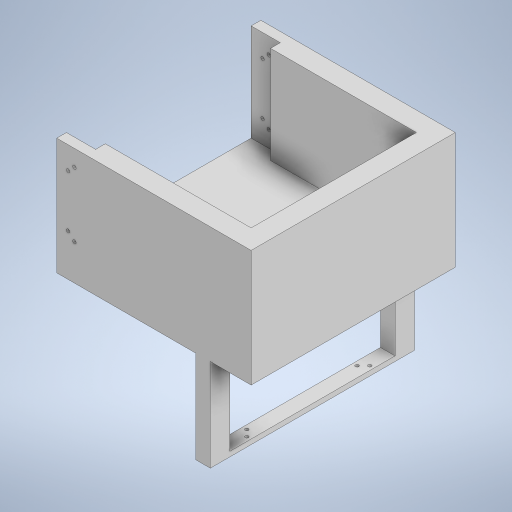
# Autodesk Inventor part: container_front
Saved by Autodesk Inventor 2023 (Build 270158000, 158)
## iProperties
Created: 2022-10-30
Part Number: container_front
Material: Genérico
Document SubType Name: Modeling
Designer: papel
Density: 1 g/cm^3
Appearance: Valor por defecto
Surface Area: 1558.19 cm^2
Author: papel
Autodesk Inventor part; units mm, degrees
ref_plane "YZ Plane" through (0, 0, 0) normal (1, 0, 0) x (0, 1, 0)
ref_plane "XZ Plane" through (0, 0, 0) normal (0, 1, 0) x (-1, 0, 0)
ref_plane "XY Plane" through (0, 0, 0) normal (0, 0, 1) x (1, 0, 0)
sketch "Boceto2" plane through (0, 0, 0) normal (0, 1, 0) x (-1, 0, 0)
  line L0 (7.5, 105) -> (-7.5, 105)
  line L1 (-7.5, 105) -> (-7.5, -105)
  line L2 (-7.5, -105) -> (7.5, -105)
  line L3 (7.5, -105) -> (7.5, 105)
  line L4 (7.5, 105) -> (-7.5, -105) construction
  line L5 (-7.5, 105) -> (7.5, -105) construction
  point P0 (0, 0)
  dimension "d7" = 15
  dimension "d8" = 210
  constraints: 12 end point, 2 midpoint, 2 parallel, 1 horizontal, 1 perpendicular
  measures "d7" distance of L2.end L1.end
  measures "d8" distance of L1.end L0.end
extrude "Extrusión1" add sketch "Boceto2" along normal blind 5
sketch "Boceto3" plane through (0, 5, 0) normal (0, 1, 0) x (1, 0, 0)
  circle A0 centre (3.25, 63.25) radius 1.75
  line L0 (5, 55) -> (-5, 55)
  line L1 (-5, 55) -> (-5, 65)
  line L2 (-5, 65) -> (5, 65)
  line L3 (5, 65) -> (5, 55)
  line L4 (5, 55) -> (-5, 65) construction
  line L5 (-5, 55) -> (5, 65) construction
  circle A1 centre (-3.25, 56.75) radius 1.75
  line L6 (7.5, 105) -> (-7.5, 105) projected
  line L7 (-7.5, 0) -> (3.408, 0)
  line L8 (5, -65) -> (5, -55)
  line L9 (-5, -65) -> (5, -65)
  line L10 (5, -55) -> (-5, -55)
  line L11 (-5, -55) -> (-5, -65)
  line L12 (-5, -55) -> (5, -65) construction
  circle A2 centre (-3.25, -56.75) radius 1.75
  line L13 (5, -55) -> (-5, -65) construction
  circle A3 centre (3.25, -63.25) radius 1.75
  point P0 (0, 0)
  point P1 (-5, 60)
  point P2 (0, 105)
  point P3 (-5, -60)
  dimension "d11" = 3.5
  dimension "d12" = 1.75
  dimension "d13" = 1.75
  dimension "d14" = 1.75
  dimension "d15" = 1.75
  dimension "d16" = 10
  dimension "d17" = 10
  dimension "d19" = 40
  constraints: 26 end point, 7 symmetric about line, 4 centre point, 2 horizontal, 2 midpoint, 2 parallel, 1 perpendicular, 2 other
  measures "d11" diameter of A0
  measures "d12" distance from line of L2 A0.centre
  measures "d13" distance from line of L3 A0.centre
  measures "d14" distance from line of L1 A1.centre
  measures "d15" distance from line of L0 A1.centre
  measures "d16" distance between parallel lines of L0 L2
  measures "d17" distance between parallel lines of L3 L1
  measures "d19" distance from line of point (0, 105) L2
hole "Agujero1" at (3.25, 5, 63.25) at (-3.25, 5, 56.75) at (3.25, 5, -63.25) at (-3.25, 5, -56.75) direction (0, -1, 0) diameter 3.5 end through all
sketch "Boceto4" plane through (0, 5, 0) normal (0, 1, 0) x (1, 0, 0)
  line L0 (-7.5, 105) -> (-7.5, -105) projected
  line L1 (-7.5, -105) -> (7.5, -105)
  line L2 (7.5, -105) -> (7.5, -85)
  line L3 (7.5, -85) -> (-7.5, -85)
  line L4 (-7.5, -85) -> (-7.5, -105)
  line L5 (-7.5, 0) -> (1.0116, 0)
  line L6 (-7.5, -105) -> (-7.5, 105)
  line L7 (-7.5, 105) -> (7.5, 105)
  line L8 (7.5, 105) -> (7.5, 85)
  line L9 (7.5, 85) -> (-7.5, 85)
  line L10 (-7.5, 85) -> (-7.5, 105)
  point P0 (0, 0)
  dimension "d27" = 15
  dimension "d28" = 20
  constraints: 20 end point, 5 symmetric about line, 2 horizontal, 2 parallel, 1 midpoint, 1 perpendicular
  measures "d27" distance of L3.end L2.end
  measures "d28" distance of L2.end L1.end
extrude "Extrusión2" add sketch "Boceto4" along normal blind 90
sketch "Boceto5" plane through (0, 95, 0) normal (0, 1, 0) x (1, 0, 0)
  line L0 (-7.5, -105) -> (7.5, -105) projected
  line L1 (-7.5, -105) -> (49.5, -105)
  line L2 (49.5, -105) -> (49.5, 105)
  line L3 (49.5, 105) -> (-7.5, 105)
  line L4 (-7.5, 105) -> (-7.5, -105)
  line L5 (49.5, -105) -> (-150.5, -105)
  line L6 (-150.5, -105) -> (-150.5, 105)
  line L7 (-150.5, 105) -> (49.5, 105)
  line L8 (49.5, 105) -> (49.5, -105)
  point P0 (0, 0)
  dimension "d31" = 57
  dimension "d32" = 200
  constraints: 16 end point, 4 parallel, 2 horizontal, 2 perpendicular, 1 point on line
  measures "d31" distance of L3.end L2.end
  measures "d32" distance of L6.end L7.end
extrude "Extrusión3" add sketch "Boceto5" along normal blind 120
sketch "Boceto6" plane through (0, 215, 0) normal (0, 1, 0) x (1, 0, 0)
  line L0 (49.5, 105) -> (7.5, 105) projected
  line L1 (49.5, 105) -> (29.5, 105)
  line L2 (29.5, 105) -> (29.5, 85)
  line L3 (7.5, -105) -> (49.5, -105) projected
  line L4 (28.5, -105) -> (28.5, -85)
  line L5 (-150.5, 105) -> (-150.5, -105) projected
  line L6 (29.5, 85) -> (-150.5, 85)
  line L7 (-150.5, 85) -> (-150.5, -85)
  line L8 (-150.5, -85) -> (29.5, -85)
  line L9 (29.5, -85) -> (29.5, 85)
  point P0 (7.5, 85)
  dimension "d36" = 20
  dimension "d37" = 20
  dimension "d38" = 20
  constraints: 14 end point, 2 parallel, 2 perpendicular, 2 point on line, 1 horizontal, 1 midpoint, 1 vertical
  measures "d36" distance of L0.start L1.end
  measures "d37" distance of L1.end L2.end
  measures "d38" distance of L4.start L4.end
extrude "Extrusión4" cut sketch "Boceto6" against normal blind 100
sketch "Boceto7" plane through (-150.5, 95, -105) normal (-1, 0, 0) x (0, 0, 1)
  line L0 (0, 120) -> (20, 120) projected
  line L1 (20, 120) -> (10, 120)
  line L2 (10, 120) -> (10, 20)
  line L3 (10, 20) -> (20, 20)
  line L4 (20, 20) -> (20, 120)
  line L5 (190, 120) -> (190, 20) projected
  line L6 (190, 120) -> (200, 120)
  line L7 (200, 120) -> (200, 20)
  line L8 (200, 20) -> (190, 20)
  line L9 (190, 20) -> (190, 120)
  line L10 (210, 0) -> (210, 120) projected
  line L11 (0, 0) -> (0, 120) projected
  line L12 (0, 120) -> (10, 120)
  line L13 (10, 120) -> (10, 20)
  line L14 (10, 20) -> (0, 20)
  line L15 (0, 20) -> (0, 120)
  line L16 (210, 120) -> (0, 120) projected
  line L17 (210, 120) -> (200, 120)
  line L18 (200, 120) -> (200, 20)
  line L19 (200, 20) -> (210, 20)
  line L20 (210, 20) -> (210, 120)
  point P0 (105, -95)
  dimension "d42" = 10
  dimension "d63" = 10
  dimension "d65" = 10
  constraints: 32 end point, 8 parallel, 4 horizontal, 4 perpendicular, 1 point on line
  measures "d42" distance of L7.end L8.end
  measures "d63" distance between parallel lines of L10 L7
  measures "d65" distance between parallel lines of L11 L2
extrude "Extrusión5" cut sketch "Boceto7" against normal blind 30 contours L0 L4 L3 L2 | L6 L7 L8 L5
sketch "Boceto8" plane through (-7.5, 0, 105) normal (0, 0, 1) x (1, 0, 0)
  line L0 (-113, 115) -> (-113, 215) projected
  line L1 (-113, 215) -> (-113, 115)
  circle A0 centre (-124.75, 198.25) radius 1.75
  line L2 (-123, 190) -> (-133, 190)
  line L3 (-133, 190) -> (-133, 200)
  line L4 (-133, 200) -> (-123, 200)
  line L5 (-123, 200) -> (-123, 190)
  line L6 (-123, 190) -> (-133, 200) construction
  line L7 (-133, 190) -> (-123, 200) construction
  circle A1 centre (-131.25, 191.75) radius 1.75
  line L8 (-143, 215) -> (57, 215) projected
  line L9 (-143, 95) -> (-143, 215) projected
  line L10 (-113, 165) -> (-128, 165)
  line L11 (-123, 130) -> (-123, 140)
  line L12 (-133, 130) -> (-123, 130)
  line L13 (-123, 140) -> (-133, 130) construction
  line L14 (-123, 140) -> (-133, 140)
  line L15 (-133, 140) -> (-123, 130) construction
  circle A2 centre (-131.25, 138.25) radius 1.75
  line L16 (-133, 140) -> (-133, 130)
  circle A3 centre (-124.75, 131.75) radius 1.75
  line L17 (-143, 115) -> (-113, 115) projected
  point P0 (7.5, 0)
  point P1 (-133, 195)
  point P2 (-123, 195)
  point P3 (-133, 135)
  point P4 (-123, 135)
  dimension "d45" = 3.5
  dimension "d46" = 1.75
  dimension "d47" = 1.75
  dimension "d48" = 1.75
  dimension "d49" = 1.75
  dimension "d50" = 10
  dimension "d51" = 10
  dimension "d52" = 15
  dimension "d53" = 10
  dimension "d54" = 10
  dimension "d55" = 15
  constraints: 28 end point, 8 symmetric about line, 4 centre point, 3 equal length, 3 midpoint, 2 horizontal, 1 perpendicular, 2 other
  measures "d45" diameter of A0
  measures "d46" distance from line of L4 A0.centre
  measures "d47" distance from line of L5 A0.centre
  measures "d48" distance from line of L3 A1.centre
  measures "d49" distance from line of L2 A1.centre
  measures "d50" distance between parallel lines of L2 L4
  measures "d51" distance between parallel lines of L5 L3
  measures "d52" distance between parallel lines of L8 L4
  measures "d53" distance between parallel lines of L9 L3
  measures "d54" distance from line of L0 point (-123, 195)
  measures "d55" distance between parallel lines of L17 L12
hole "Agujero2" at (-132.25, 198.25, 105) at (-138.75, 191.75, 105) at (-138.75, 138.25, 105) at (-132.25, 131.75, 105) direction (0, 0, -1) diameter 3.5 end through all
